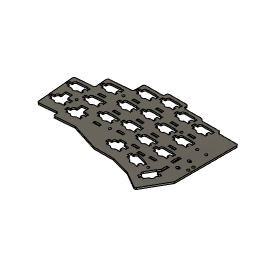
BottomCutout (Autodesk Fusion 360 design; units mm, degrees)
Autodesk Fusion 360 part; units mm, degrees
sketch "bottom-cutout-Edge_Cuts" plane through (0, 0, 0) normal (0, 0, 1) x (1, 0, 0)
  line L0 (132.25, -118) -> (132.25, -116)
  line L1 (110.25, -54.5) -> (110.25, -56.5)
  line L2 (121.75, -51.75) -> (124.5, -51.75)
  line L3 (121.75, -54.5) -> (121.75, -51.75)
  line L4 (130.75, -110.5) -> (130.75, -110)
  line L5 (140.75, -53.5) -> (140.75, -53)
  line L6 (126.75, -59) -> (129.25, -59)
  arc A0 (131.464, -53) -> (129.4503, -54.9213) centre (131.464, -55.016) ccw
  line L7 (121.75, -86.5) -> (112.464, -86.5)
  line L8 (123.25, -92.5) -> (121.75, -92.5)
  line L9 (129.45, -56) -> (129.45, -54.9321)
  line L10 (121.75, -92.5) -> (121.75, -89.75)
  line L11 (110.45, -89.5) -> (110.45, -88.4314)
  line L12 (129.25, -59) -> (129.25, -61)
  arc A1 (70.6704, -64.8002) -> (68.832, -66.8948) centre (70.8461, -66.8085) ccw
  line L13 (140.75, -53) -> (131.464, -53)
  arc A2 (73.5435, -72.8271) -> (77.7738, -72.457) centre (75.55, -71.4) ccw
  line L14 (66.2356, -68.1996) -> (66.4971, -71.1882)
  line L15 (142.25, -61) -> (142.25, -59)
  line L16 (124.5, -87) -> (121.75, -87)
  arc A3 (133.6268, -61.2468) -> (137.8732, -61.2468) centre (135.75, -60) ccw
  line L17 (123.25, -94.5) -> (123.25, -92.5)
  line L18 (140.75, -59) -> (140.75, -56.25)
  line L19 (143.5, -56.25) -> (143.5, -53.5)
  line L20 (138.3044, -61) -> (142.25, -61)
  line L21 (124.5, -89.75) -> (124.5, -87)
  line L22 (119.361, -94.5) -> (123.25, -94.5)
  line L23 (129.45, -56) -> (126.75, -56)
  line L24 (107.75, -92.5) -> (110.25, -92.5)
  line L25 (142.25, -59) -> (140.75, -59)
  line L26 (121.75, -89.75) -> (124.5, -89.75)
  line L27 (110.45, -89.5) -> (107.75, -89.5)
  line L28 (140.75, -56.25) -> (143.5, -56.25)
  line L29 (143.5, -53.5) -> (140.75, -53.5)
  line L30 (110.25, -94.5) -> (114.139, -94.5)
  line L31 (110.25, -56.5) -> (114.139, -56.5)
  arc A4 (114.6506, -94.7865) -> (118.8494, -94.7865) centre (116.75, -93.5) ccw
  line L32 (110.45, -51.5) -> (110.45, -50.4314)
  line L33 (124.5, -51.75) -> (124.5, -49)
  line L34 (119.45, -113) -> (116.75, -113)
  line L35 (116.75, -113) -> (116.75, -116)
  arc A5 (123.6268, -118.2468) -> (127.8732, -118.2468) centre (125.75, -117) ccw
  line L36 (133.5, -113.25) -> (133.5, -110.5)
  line L37 (121.75, -48.5) -> (112.464, -48.5)
  line L38 (128.3044, -118) -> (132.25, -118)
  line L39 (110.45, -51.5) -> (107.75, -51.5)
  line L40 (124.5, -49) -> (121.75, -49)
  line L41 (123.25, -56.5) -> (123.25, -54.5)
  line L42 (121.75, -87) -> (121.75, -86.5)
  line L43 (130.75, -116) -> (130.75, -113.25)
  line L44 (119.25, -118) -> (123.1956, -118)
  line L45 (119.25, -116) -> (119.25, -118)
  line L46 (133.5, -110.5) -> (130.75, -110.5)
  line L47 (132.25, -116) -> (130.75, -116)
  arc A6 (112.464, -86.5) -> (110.4502, -88.4221) centre (112.464, -88.516) ccw
  line L48 (107.75, -89.5) -> (107.75, -92.5)
  line L49 (130.75, -113.25) -> (133.5, -113.25)
  line L50 (119.45, -113) -> (119.45, -111.9321)
  arc A7 (121.464, -110) -> (119.4503, -111.9213) centre (121.464, -112.016) ccw
  line L51 (116.75, -116) -> (119.25, -116)
  line L52 (123.25, -54.5) -> (121.75, -54.5)
  line L53 (107.75, -51.5) -> (107.75, -54.5)
  arc A8 (112.464, -48.5) -> (110.4502, -50.4221) centre (112.464, -50.516) ccw
  line L54 (107.75, -54.5) -> (110.25, -54.5)
  line L55 (121.75, -49) -> (121.75, -48.5)
  arc A9 (114.6506, -56.7865) -> (118.8494, -56.7865) centre (116.75, -55.5) ccw
  line L56 (119.361, -56.5) -> (123.25, -56.5)
  line L57 (138.565, -116.455) -> (140.98, -117.102)
  line L58 (139.342, -113.557) -> (138.565, -116.455)
  line L59 (68.9253, -67.9643) -> (66.2356, -68.1996)
  line L60 (152.088, -120.078) -> (152.8, -117.422)
  line L61 (141.95, -114.256) -> (142.2254, -113.2276)
  line L62 (82.1124, -71.8297) -> (81.9381, -69.8373)
  line L63 (153.641, -114.283) -> (144.6718, -111.8797)
  line L64 (80.2041, -67.2285) -> (82.9437, -66.9888)
  line L65 (140.463, -119.034) -> (144.274, -120.0552)
  arc A10 (144.6265, -120.4051) -> (148.7284, -121.5036) centre (147, -119.75) ccw
  line L66 (78.1818, -72.1736) -> (82.1124, -71.8297)
  line L67 (152.8, -117.422) -> (155.456, -118.134)
  line L68 (79.9645, -64.489) -> (79.9209, -63.9909)
  line L69 (68.9253, -67.9643) -> (68.8326, -66.9036)
  line L70 (156.168, -115.477) -> (153.512, -114.766)
  arc A11 (75.1935, -91.7771) -> (79.4238, -91.407) centre (77.2, -90.35) ccw
  line L71 (141.95, -114.256) -> (139.342, -113.557)
  line L72 (140.98, -117.102) -> (140.463, -119.034)
  line L73 (81.9381, -69.8373) -> (80.4438, -69.968)
  line L74 (69.1619, -72.9627) -> (73.0925, -72.6188)
  line L75 (110.25, -92.5) -> (110.25, -94.5)
  line L76 (82.9437, -66.9888) -> (82.704, -64.2493)
  line L77 (153.537, -120.466) -> (152.088, -120.078)
  line L78 (129.25, -61) -> (133.1956, -61)
  line L79 (155.456, -118.134) -> (156.168, -115.477)
  arc A12 (144.6718, -111.8797) -> (142.2284, -113.2175) centre (144.15, -113.827) ccw
  line L80 (126.75, -56) -> (126.75, -59)
  line L81 (91.45, -74.5) -> (91.45, -73.4365)
  line L82 (104.25, -77.5) -> (102.75, -77.5)
  line L83 (102.75, -72) -> (102.75, -71.5)
  line L84 (88.75, -74.5) -> (88.75, -77.5)
  line L85 (100.3044, -79.5) -> (104.25, -79.5)
  line L86 (91.25, -77.5) -> (91.25, -79.5)
  arc A13 (93.4642, -71.5) -> (91.4502, -73.4263) centre (93.4642, -73.516) ccw
  line L87 (62.0819, -106.3735) -> (66.0124, -106.03)
  line L88 (50.1356, -102.4) -> (50.3971, -105.388)
  arc A14 (95.6268, -79.7468) -> (99.8732, -79.7468) centre (97.75, -78.5) ccw
  line L89 (63.8645, -98.689) -> (63.8209, -98.1909)
  line L90 (105.5, -74.75) -> (105.5, -72)
  line L91 (66.604, -98.4493) -> (63.8645, -98.689)
  line L92 (91.25, -79.5) -> (95.1956, -79.5)
  line L93 (51.1253, -83.1643) -> (48.4356, -83.3996)
  line L94 (104.25, -79.5) -> (104.25, -77.5)
  line L95 (102.75, -71.5) -> (93.4642, -71.5)
  arc A15 (54.5221, -99.0045) -> (52.7321, -101.0967) centre (54.7461, -101.008) ccw
  line L96 (66.8437, -101.189) -> (66.604, -98.4493)
  line L97 (88.75, -77.5) -> (91.25, -77.5)
  line L98 (66.0124, -106.03) -> (65.8381, -104.037)
  line L99 (52.8876, -105.17) -> (53.0619, -107.163)
  line L100 (64.3438, -104.168) -> (64.1041, -101.428)
  line L101 (102.75, -77.5) -> (102.75, -74.75)
  arc A16 (57.4434, -107.0269) -> (61.6738, -106.657) centre (59.45, -105.6) ccw
  line L102 (65.8381, -104.037) -> (64.3438, -104.168)
  line L103 (52.8254, -102.164) -> (52.7327, -101.1054)
  line L104 (50.3971, -105.388) -> (52.8876, -105.17)
  line L105 (91.45, -74.5) -> (88.75, -74.5)
  line L106 (48.4356, -83.3996) -> (48.6971, -86.3882)
  line L107 (60.4382, -87.3686) -> (64.3124, -87.0297)
  line L108 (62.6438, -85.168) -> (62.4041, -82.4285)
  line L109 (65.1437, -82.1888) -> (64.904, -79.4493)
  line L110 (105.5, -72) -> (102.75, -72)
  line L111 (102.75, -74.75) -> (105.5, -74.75)
  line L112 (70.6376, -89.9203) -> (70.8119, -91.9127)
  line L113 (68.1471, -90.1382) -> (70.6376, -89.9203)
  line L114 (81.5709, -82.9409) -> (72.3204, -83.7502)
  arc A17 (72.3204, -83.7502) -> (70.482, -85.8452) centre (72.4961, -85.7585) ccw
  line L115 (81.6145, -83.439) -> (81.5709, -82.9409)
  line L116 (67.8856, -87.1496) -> (68.1471, -90.1382)
  line L117 (83.5881, -88.7873) -> (82.0938, -88.918)
  line L118 (48.6971, -86.3882) -> (51.1876, -86.1703)
  line L119 (83.7624, -90.7797) -> (83.5881, -88.7873)
  line L120 (62.1209, -79.1909) -> (52.8704, -80.0002)
  arc A18 (52.8704, -80.0002) -> (51.0319, -82.094) centre (53.0461, -82.0085) ccw
  line L121 (64.1381, -85.0373) -> (62.6438, -85.168)
  line L122 (82.0938, -88.918) -> (81.8541, -86.1785)
  line L123 (64.904, -79.4493) -> (62.1645, -79.689)
  line L124 (70.5754, -86.9143) -> (67.8856, -87.1496)
  line L125 (70.5754, -86.9143) -> (70.4826, -85.8541)
  line L126 (81.8541, -86.1785) -> (84.5937, -85.9388)
  line L127 (62.4041, -82.4285) -> (65.1437, -82.1888)
  line L128 (51.1253, -83.1643) -> (51.0326, -82.1043)
  line L129 (79.8318, -91.1236) -> (83.7624, -90.7797)
  line L130 (62.1645, -79.689) -> (62.1209, -79.1909)
  line L131 (70.8119, -91.9127) -> (74.7425, -91.5688)
  arc A19 (55.7707, -88.0646) -> (59.9535, -87.6986) centre (57.75, -86.6) ccw
  line L132 (51.3619, -88.1627) -> (55.2361, -87.8238)
  line L133 (84.5937, -85.9388) -> (84.354, -83.1993)
  line L134 (64.3124, -87.0297) -> (64.1381, -85.0373)
  line L135 (84.354, -83.1993) -> (81.6145, -83.439)
  line L136 (66.4971, -71.1882) -> (68.9876, -70.9703)
  line L137 (80.4438, -69.968) -> (80.2041, -67.2285)
  line L138 (68.9876, -70.9703) -> (69.1619, -72.9627)
  line L139 (79.9209, -63.9909) -> (70.6704, -64.8002)
  line L140 (153.512, -114.766) -> (153.641, -114.283)
  line L141 (82.704, -64.2493) -> (79.9645, -64.489)
  line L142 (153.02, -122.398) -> (153.537, -120.466)
  line L143 (149.2088, -121.3767) -> (153.02, -122.398)
  line L144 (51.1876, -86.1703) -> (51.3619, -88.1627)
  line L145 (141.75, -110.5) -> (147.75, -110.5)
  line L146 (100.75, -66.5) -> (94.75, -66.5)
  line L147 (80.7046, -97.0396) -> (74.7275, -97.5625)
  line L148 (132.75, -69.0483) -> (138.75, -69.0483)
  line L149 (74.7275, -97.5625) -> (75.1678, -102.5953)
  line L150 (61.4514, -93.3423) -> (55.4743, -93.8653)
  line L151 (138.75, -105.048) -> (132.75, -105.048)
  line L152 (132.75, -67.0483) -> (132.75, -69.0483)
  line L153 (141.75, -108.5) -> (141.75, -110.5)
  line L154 (167.95, -107.3) -> (169.95, -107.3)
  line L155 (55.4743, -93.8653) -> (55.9132, -98.8827)
  line L156 (138.75, -67.0483) -> (132.75, -67.0483)
  line L157 (132.75, -88.0483) -> (138.75, -88.0483)
  line L158 (119.75, -62.5) -> (113.75, -62.5)
  line L159 (61.8903, -98.3598) -> (61.4514, -93.3423)
  line L160 (94.75, -87.5) -> (100.75, -87.5)
  arc A20 (175.35, -104.55) -> (175.35, -102.15) centre (175.35, -103.35) ccw
  line L161 (94.75, -104.5) -> (94.75, -106.5)
  line L162 (94.75, -68.5) -> (100.75, -68.5)
  line L163 (100.75, -106.5) -> (100.75, -104.5)
  line L164 (151.75, -109) -> (157.75, -109)
  line L165 (94.75, -106.5) -> (100.75, -106.5)
  line L166 (100.75, -87.5) -> (100.75, -85.5)
  circle A21 centre (181.75, -95.25) radius 1.25
  line L167 (100.75, -104.5) -> (94.75, -104.5)
  line L168 (151.75, -88) -> (151.75, -90)
  line L169 (138.75, -86.0483) -> (132.75, -86.0483)
  line L170 (132.75, -86.0483) -> (132.75, -88.0483)
  line L171 (151.75, -107) -> (151.75, -109)
  line L172 (94.75, -85.5) -> (94.75, -87.5)
  line L173 (128.75, -107.5) -> (122.75, -107.5)
  line L174 (173.366, -118.371) -> (171.634, -117.371)
  line L175 (163.884, -130.794) -> (165.134, -128.629)
  line L176 (138.75, -88.0483) -> (138.75, -86.0483)
  line L177 (128.75, -110) -> (128.75, -107.5)
  line L178 (157.75, -90) -> (157.75, -88)
  line L179 (151.75, -90) -> (157.75, -90)
  line L180 (122.75, -107.5) -> (122.75, -110)
  line L181 (119.75, -102.5) -> (119.75, -100.5)
  line L182 (113.75, -62.5) -> (113.75, -64.5)
  line L183 (151.75, -71) -> (157.75, -71)
  line L184 (157.75, -71) -> (157.75, -69)
  line L185 (157.75, -109) -> (157.75, -107)
  line L186 (119.75, -64.5) -> (119.75, -62.5)
  line L187 (157.75, -107) -> (151.75, -107)
  line L188 (113.75, -64.5) -> (119.75, -64.5)
  line L189 (157.75, -88) -> (151.75, -88)
  line L190 (157.75, -69) -> (151.75, -69)
  line L191 (151.75, -69) -> (151.75, -71)
  line L192 (170.884, -118.67) -> (168.502, -117.295)
  line L193 (168.502, -117.295) -> (169.95, -114.7865)
  line L194 (100.361, -60.5) -> (104.25, -60.5)
  line L195 (119.75, -100.5) -> (113.75, -100.5)
  line L196 (88.75, -58.5) -> (91.25, -58.5)
  line L197 (167.95, -112.7515) -> (166.121, -115.92)
  line L198 (79.223, -80.1043) -> (79.0487, -78.1119)
  line L199 (91.45, -93.5) -> (91.45, -92.4358)
  line L200 (104.25, -60.5) -> (104.25, -58.5)
  line L201 (102.75, -96.5) -> (102.75, -93.75)
  line L202 (91.45, -55.5) -> (91.45, -54.4358)
  line L203 (165.688, -115.67) -> (161.045, -123.712)
  line L204 (161.286, -129.294) -> (163.884, -130.794)
  line L205 (166.121, -115.92) -> (165.688, -115.67)
  arc A22 (95.6506, -60.7865) -> (99.8494, -60.7865) centre (97.75, -59.5) ccw
  line L206 (91.45, -93.5) -> (88.75, -93.5)
  line L207 (102.75, -53) -> (102.75, -52.5)
  line L208 (102.75, -55.75) -> (105.5, -55.75)
  line L209 (113.75, -100.5) -> (113.75, -102.5)
  line L210 (171.634, -117.371) -> (170.884, -118.67)
  line L211 (113.75, -83.5) -> (119.75, -83.5)
  line L212 (79.0487, -78.1119) -> (73.0715, -78.6348)
  line L213 (166.866, -129.629) -> (168.8391, -126.2121)
  line L214 (119.75, -83.5) -> (119.75, -81.5)
  line L215 (105.5, -93.75) -> (105.5, -91)
  line L216 (113.75, -81.5) -> (113.75, -83.5)
  line L217 (104.25, -98.5) -> (104.25, -96.5)
  line L218 (100.361, -98.5) -> (104.25, -98.5)
  line L219 (91.25, -98.5) -> (95.139, -98.5)
  line L220 (119.75, -81.5) -> (113.75, -81.5)
  line L221 (113.75, -102.5) -> (119.75, -102.5)
  line L222 (171.3931, -121.7876) -> (173.366, -118.371)
  line L223 (162.636, -126.956) -> (161.286, -129.294)
  line L224 (102.75, -58.5) -> (102.75, -55.75)
  line L225 (102.75, -52.5) -> (93.4642, -52.5)
  line L226 (88.75, -55.5) -> (88.75, -58.5)
  line L227 (104.25, -58.5) -> (102.75, -58.5)
  line L228 (73.0715, -78.6348) -> (73.2458, -80.6272)
  line L229 (73.2458, -80.6272) -> (79.223, -80.1043)
  line L230 (102.75, -90.5) -> (93.4642, -90.5)
  line L231 (91.45, -55.5) -> (88.75, -55.5)
  line L232 (91.25, -58.5) -> (91.25, -60.5)
  arc A23 (161.045, -123.712) -> (161.7079, -126.4203) centre (162.7911, -124.7199) ccw
  line L233 (105.5, -55.75) -> (105.5, -53)
  line L234 (105.5, -53) -> (102.75, -53)
  line L235 (102.75, -93.75) -> (105.5, -93.75)
  line L236 (91.25, -96.5) -> (91.25, -98.5)
  line L237 (165.134, -128.629) -> (166.866, -129.629)
  arc A24 (169.2683, -125.9621) -> (171.3913, -122.2845) centre (169.25, -123.5) ccw
  line L238 (104.25, -96.5) -> (102.75, -96.5)
  arc A25 (95.6506, -98.7865) -> (99.8494, -98.7865) centre (97.75, -97.5) ccw
  line L239 (105.5, -91) -> (102.75, -91)
  line L240 (162.636, -126.956) -> (161.7165, -126.4255)
  line L241 (91.25, -60.5) -> (95.139, -60.5)
  arc A26 (93.4642, -52.5) -> (91.4502, -54.427) centre (93.4642, -54.516) ccw
  line L242 (86.004, -102.149) -> (83.2645, -102.389)
  line L243 (159.75, -74) -> (150.464, -74)
  line L244 (88.75, -93.5) -> (88.75, -96.5)
  line L245 (148.25, -82) -> (152.139, -82)
  line L246 (143.5, -94.25) -> (143.5, -91.5)
  arc A27 (93.4642, -90.5) -> (91.4502, -92.427) centre (93.4642, -92.516) ccw
  line L247 (140.75, -91) -> (131.464, -91)
  arc A28 (133.6506, -99.2865) -> (137.8494, -99.2865) centre (135.75, -98) ccw
  arc A29 (152.6506, -82.2865) -> (156.8494, -82.2865) centre (154.75, -81) ccw
  line L248 (148.25, -80) -> (148.25, -82)
  line L249 (143.5, -91.5) -> (140.75, -91.5)
  line L250 (159.75, -61) -> (159.75, -58.25)
  line L251 (148.25, -63) -> (152.139, -63)
  arc A30 (76.8434, -110.7269) -> (81.0738, -110.357) centre (78.85, -109.3) ccw
  line L252 (72.4619, -110.863) -> (76.3923, -110.5186)
  line L253 (69.5356, -106.1) -> (69.7971, -109.088)
  arc A31 (73.9307, -102.7036) -> (72.132, -104.7955) centre (74.1461, -104.708) ccw
  line L254 (145.75, -80) -> (148.25, -80)
  line L255 (161.25, -80) -> (159.75, -80)
  arc A32 (131.464, -91) -> (129.4502, -92.9221) centre (131.464, -93.016) ccw
  line L256 (148.25, -61) -> (148.25, -63)
  line L257 (148.45, -77) -> (145.75, -77)
  line L258 (129.45, -94) -> (126.75, -94)
  line L259 (129.45, -94) -> (129.45, -92.9314)
  line L260 (159.75, -74.5) -> (159.75, -74)
  line L261 (140.75, -91.5) -> (140.75, -91)
  line L262 (159.75, -77.25) -> (162.5, -77.25)
  line L263 (69.7971, -109.088) -> (72.2876, -108.87)
  line L264 (86.2437, -104.889) -> (86.004, -102.149)
  line L265 (83.2645, -102.389) -> (83.2209, -101.891)
  line L266 (161.25, -82) -> (161.25, -80)
  line L267 (159.75, -58.25) -> (162.5, -58.25)
  line L268 (140.75, -78) -> (140.75, -75.25)
  line L269 (140.75, -97) -> (140.75, -94.25)
  line L270 (148.45, -58) -> (145.75, -58)
  line L271 (162.5, -74.5) -> (159.75, -74.5)
  line L272 (148.45, -58) -> (148.45, -56.9314)
  arc A33 (150.464, -74) -> (148.4502, -75.9221) centre (150.464, -76.016) ccw
  line L273 (72.2876, -108.87) -> (72.4619, -110.863)
  line L274 (157.361, -82) -> (161.25, -82)
  line L275 (129.25, -99) -> (133.139, -99)
  line L276 (159.75, -80) -> (159.75, -77.25)
  line L277 (126.75, -94) -> (126.75, -97)
  line L278 (142.25, -97) -> (140.75, -97)
  line L279 (88.75, -96.5) -> (91.25, -96.5)
  line L280 (83.5041, -105.128) -> (86.2437, -104.889)
  line L281 (145.75, -77) -> (145.75, -80)
  line L282 (83.7438, -107.868) -> (83.5041, -105.128)
  line L283 (85.2381, -107.737) -> (83.7438, -107.868)
  line L284 (138.361, -99) -> (142.25, -99)
  line L285 (162.5, -77.25) -> (162.5, -74.5)
  line L286 (129.25, -97) -> (129.25, -99)
  line L287 (142.25, -99) -> (142.25, -97)
  line L288 (126.75, -97) -> (129.25, -97)
  line L289 (140.75, -94.25) -> (143.5, -94.25)
  line L290 (72.2253, -105.864) -> (72.1327, -104.8056)
  line L291 (148.45, -77) -> (148.45, -75.9314)
  line L292 (159.75, -55) -> (150.464, -55)
  line L293 (85.4124, -109.73) -> (85.2381, -107.737)
  line L294 (81.4819, -110.0735) -> (85.4124, -109.73)
  line L295 (72.2253, -105.864) -> (69.5356, -106.1)
  line L296 (102.75, -91) -> (102.75, -90.5)
  line L297 (148.45, -96) -> (145.75, -96)
  line L298 (143.5, -72.5) -> (140.75, -72.5)
  line L299 (124.5, -68) -> (121.75, -68)
  line L300 (110.45, -70.5) -> (110.45, -69.4314)
  line L301 (145.75, -96) -> (145.75, -99)
  line L302 (121.75, -67.5) -> (112.464, -67.5)
  arc A34 (114.6506, -75.7865) -> (118.8494, -75.7865) centre (116.75, -74.5) ccw
  line L303 (140.75, -72.5) -> (140.75, -72)
  line L304 (140.75, -72) -> (131.464, -72)
  line L305 (148.45, -96) -> (148.45, -94.9314)
  line L306 (159.75, -99) -> (159.75, -96.25)
  arc A35 (112.464, -67.5) -> (110.4502, -69.4221) centre (112.464, -69.516) ccw
  arc A36 (150.464, -55) -> (148.4502, -56.9221) centre (150.464, -57.016) ccw
  line L307 (129.25, -78) -> (129.25, -80)
  line L308 (143.5, -75.25) -> (143.5, -72.5)
  line L309 (148.25, -101) -> (152.139, -101)
  line L310 (123.25, -73.5) -> (121.75, -73.5)
  line L311 (145.75, -99) -> (148.25, -99)
  arc A37 (152.6506, -63.2865) -> (156.8494, -63.2865) centre (154.75, -62) ccw
  line L312 (157.361, -101) -> (161.25, -101)
  line L313 (148.25, -99) -> (148.25, -101)
  line L314 (142.25, -80) -> (142.25, -78)
  line L315 (110.45, -70.5) -> (107.75, -70.5)
  line L316 (121.75, -70.75) -> (124.5, -70.75)
  line L317 (142.25, -78) -> (140.75, -78)
  line L318 (162.5, -58.25) -> (162.5, -55.5)
  line L319 (107.75, -73.5) -> (110.25, -73.5)
  line L320 (162.5, -96.25) -> (162.5, -93.5)
  line L321 (53.0619, -107.163) -> (56.9923, -106.8186)
  arc A38 (133.6506, -80.2865) -> (137.8494, -80.2865) centre (135.75, -79) ccw
  line L322 (119.361, -75.5) -> (123.25, -75.5)
  line L323 (129.25, -80) -> (133.139, -80)
  arc A39 (152.6506, -101.2865) -> (156.8494, -101.2865) centre (154.75, -100) ccw
  line L324 (145.75, -61) -> (148.25, -61)
  line L325 (138.361, -80) -> (142.25, -80)
  line L326 (129.45, -75) -> (129.45, -73.9314)
  line L327 (110.25, -73.5) -> (110.25, -75.5)
  line L328 (159.75, -55.5) -> (159.75, -55)
  line L329 (162.5, -55.5) -> (159.75, -55.5)
  line L330 (145.75, -58) -> (145.75, -61)
  line L331 (121.75, -73.5) -> (121.75, -70.75)
  line L332 (124.5, -70.75) -> (124.5, -68)
  line L333 (110.25, -75.5) -> (114.139, -75.5)
  line L334 (157.361, -63) -> (161.25, -63)
  line L335 (159.75, -93.5) -> (159.75, -93)
  line L336 (52.8254, -102.164) -> (50.1356, -102.4)
  line L337 (161.25, -101) -> (161.25, -99)
  line L338 (140.75, -75.25) -> (143.5, -75.25)
  line L339 (159.75, -93) -> (150.464, -93)
  line L340 (161.25, -99) -> (159.75, -99)
  line L341 (107.75, -70.5) -> (107.75, -73.5)
  line L342 (121.75, -68) -> (121.75, -67.5)
  line L343 (64.1041, -101.428) -> (66.8437, -101.189)
  line L344 (126.75, -75) -> (126.75, -78)
  line L345 (161.25, -63) -> (161.25, -61)
  arc A40 (150.464, -93) -> (148.4502, -94.9221) centre (150.464, -95.016) ccw
  line L346 (161.25, -61) -> (159.75, -61)
  line L347 (129.45, -75) -> (126.75, -75)
  line L348 (126.75, -78) -> (129.25, -78)
  line L349 (123.25, -75.5) -> (123.25, -73.5)
  line L350 (159.75, -96.25) -> (162.5, -96.25)
  line L351 (162.5, -93.5) -> (159.75, -93.5)
  arc A41 (131.464, -72) -> (129.4502, -73.9221) centre (131.464, -74.016) ccw
  line L352 (171.2979, -140.4529) -> (184.75, -117)
  line L353 (126.75, -48.5) -> (126.75, -47)
  arc A42 (69.3738, -116.3496) -> (67.7866, -114.9968) centre (67.8807, -116.494) ccw
  arc A43 (126.75, -47) -> (125.25, -45.5) centre (125.25, -47) ccw
  line L354 (89.25, -49.5) -> (105.25, -49.5)
  line L355 (86.288, -60.3907) -> (66.1036, -62.1006)
  line L356 (64.7491, -63.7144) -> (65.6216, -74.1884)
  line L357 (169.2522, -141.0013) -> (153.75, -132)
  circle A44 centre (181.75, -100.25) radius 1.25
  arc A45 (145.75, -51) -> (144.25, -50) centre (144.25, -51.625) ccw
  line L358 (174.15, -102.15) -> (175.35, -102.15)
  line L359 (125.25, -45.5) -> (108.25, -45.5)
  line L360 (174.15, -93.35) -> (175.35, -93.35)
  line L361 (128.25, -50) -> (144.25, -50)
  line L362 (168.5, -101.5) -> (166, -101.5)
  line L363 (135.3, -127) -> (116.25, -127)
  arc A46 (174.15, -102.15) -> (174.15, -104.55) centre (174.15, -103.35) ccw
  arc A47 (164.75, -53.25) -> (163.25, -52) centre (163.25, -53.525) ccw
  line L364 (64.2789, -75.7974) -> (48.2528, -77.2764)
  line L365 (168.5, -94) -> (168.5, -101.5)
  arc A48 (175.35, -93.35) -> (175.35, -90.95) centre (175.35, -92.15) ccw
  arc A49 (184.75, -56) -> (183.25, -54.5) centre (183.25, -56) ccw
  line L366 (166, -94) -> (168.5, -94)
  line L367 (183.25, -54.5) -> (166.25, -54.5)
  circle A50 centre (87.05, -69) radius 1.15
  line L368 (94.75, -66.5) -> (94.75, -68.5)
  line L369 (147.75, -108.5) -> (141.75, -108.5)
  line L370 (174.15, -104.55) -> (175.35, -104.55)
  arc A51 (69.5512, -118.8107) -> (70.9203, -120.0986) centre (70.9992, -118.643) ccw
  arc A52 (174.15, -90.95) -> (174.15, -93.35) centre (174.15, -92.15) ccw
  line L371 (174.15, -90.95) -> (175.35, -90.95)
  arc A53 (169.2541, -141.0024) -> (171.2967, -140.455) centre (170, -139.701) ccw
  line L372 (147.75, -110.5) -> (147.75, -108.5)
  line L373 (147.25, -52) -> (163.25, -52)
  circle A54 centre (108.25, -103.5) radius 1.15
  line L374 (46.9043, -78.8946) -> (50.125, -115.082)
  circle A55 centre (159.75, -117.5) radius 1.15
  line L375 (106.75, -47) -> (106.75, -48)
  line L376 (184.75, -87) -> (184.75, -117)
  line L377 (169.95, -107.3) -> (169.95, -114.7865)
  line L378 (167.95, -112.7515) -> (167.95, -107.3)
  line L379 (100.75, -85.5) -> (94.75, -85.5)
  circle A56 centre (67.5, -95.25) radius 1.15
  arc A57 (89.25, -49.5) -> (87.75, -51) centre (89.25, -51) ccw
  circle A58 centre (146.25, -71.5) radius 1.15
  line L380 (100.75, -68.5) -> (100.75, -66.5)
  arc A59 (145.75, -51) -> (147.25, -52) centre (147.25, -50.375) ccw
  line L381 (132.75, -105.048) -> (132.75, -107.048)
  line L382 (138.75, -107.048) -> (138.75, -105.048)
  line L383 (51.7337, -116.4465) -> (67.7757, -114.9977)
  circle A60 centre (168.75, -78.5) radius 1.15
  arc A61 (48.2497, -77.2767) -> (46.9041, -78.8919) centre (48.3991, -78.7693) ccw
  circle A62 centre (177.5, -78.5) radius 1.15
  line L384 (166, -101.5) -> (166, -94)
  line L385 (69.3747, -116.3594) -> (69.5495, -118.7934)
  line L386 (81.1449, -102.0726) -> (80.7046, -97.0396)
  line L387 (138.75, -69.0483) -> (138.75, -67.0483)
  line L388 (132.75, -107.048) -> (138.75, -107.048)
  arc A63 (126.75, -48.5) -> (128.25, -50) centre (128.25, -48.5) ccw
  arc A64 (64.2839, -75.7969) -> (65.6218, -74.1912) centre (64.126, -74.3051) ccw
  line L389 (184.75, -87) -> (184.75, -56)
  arc A65 (66.0984, -62.1011) -> (64.749, -63.7128) centre (66.2444, -63.5941) ccw
  arc A66 (86.31, -60.3883) -> (87.75, -58.75) centre (86.098, -58.75) ccw
  line L390 (135.3, -127) -> (153.75, -132)
  arc A67 (164.75, -53.25) -> (166.25, -54.5) centre (166.25, -52.975) ccw
  arc A68 (108.25, -45.5) -> (106.75, -47) centre (108.25, -47) ccw
  line L391 (89.25, -118.5) -> (116.25, -127)
  line L392 (87.75, -51) -> (87.75, -58.75)
  line L393 (70.9768, -120.0977) -> (89.25, -118.5)
  arc A69 (50.125, -115.082) -> (51.7263, -116.4471) centre (51.6192, -114.951) ccw
  arc A70 (105.25, -49.5) -> (106.75, -48) centre (105.25, -48) ccw
  line L394 (63.8209, -98.1909) -> (61.8903, -98.3598)
  line L395 (55.9132, -98.8827) -> (54.5293, -99.0038)
  arc A71 (57.4434, -107.0269) -> (56.9923, -106.8186) centre (57.0359, -107.3167) ccw
  arc A72 (62.0819, -106.3735) -> (61.6738, -106.657) centre (62.1254, -106.8716) ccw
  arc A73 (54.5293, -99.0038) -> (54.5221, -99.0045) centre (54.5554, -99.3027) ccw
  arc A74 (52.7321, -101.0967) -> (52.7327, -101.1054) centre (52.9319, -101.0879) ccw
  line L396 (83.2209, -101.891) -> (81.1449, -102.0726)
  line L397 (75.1678, -102.5953) -> (73.9406, -102.7026)
  arc A75 (76.8434, -110.7269) -> (76.3923, -110.5186) centre (76.4359, -111.0167) ccw
  arc A76 (81.4819, -110.0735) -> (81.0738, -110.357) centre (81.5254, -110.5716) ccw
  arc A77 (73.9406, -102.7026) -> (73.9307, -102.7036) centre (73.9841, -103.2007) ccw
  arc A78 (72.132, -104.7955) -> (72.1327, -104.8056) centre (72.3618, -104.7856) ccw
  arc A79 (51.0319, -82.094) -> (51.0326, -82.1043) centre (51.2617, -82.0843) ccw
  arc A80 (55.7707, -88.0646) -> (55.2361, -87.8238) centre (55.2884, -88.4215) ccw
  arc A81 (60.4382, -87.3686) -> (59.9535, -87.6986) centre (60.4905, -87.9664) ccw
  arc A82 (75.1935, -91.7771) -> (74.7425, -91.5688) centre (74.7861, -92.0669) ccw
  arc A83 (79.8318, -91.1236) -> (79.4238, -91.407) centre (79.8754, -91.6217) ccw
  arc A84 (70.482, -85.8452) -> (70.4826, -85.8541) centre (70.6818, -85.8366) ccw
  arc A85 (73.5435, -72.8271) -> (73.0925, -72.6188) centre (73.1361, -73.1169) ccw
  arc A86 (78.1818, -72.1736) -> (77.7738, -72.457) centre (78.2254, -72.6717) ccw
  arc A87 (68.832, -66.8948) -> (68.8326, -66.9036) centre (69.0318, -66.8862) ccw
  arc A88 (95.6268, -79.7468) -> (95.1956, -79.5) centre (95.1956, -80) ccw
  arc A89 (100.3044, -79.5) -> (99.8732, -79.7468) centre (100.3044, -80) ccw
  arc A90 (91.4502, -73.4263) -> (91.45, -73.4365) centre (91.68, -73.4365) ccw
  arc A91 (95.6506, -98.7865) -> (95.139, -98.5) centre (95.139, -99.1) ccw
  arc A92 (100.361, -98.5) -> (99.8494, -98.7865) centre (100.361, -99.1) ccw
  arc A93 (91.4502, -92.427) -> (91.45, -92.4358) centre (91.65, -92.4358) ccw
  arc A94 (123.6268, -118.2468) -> (123.1956, -118) centre (123.1956, -118.5) ccw
  arc A95 (128.3044, -118) -> (127.8732, -118.2468) centre (128.3044, -118.5) ccw
  arc A96 (119.4503, -111.9213) -> (119.45, -111.9321) centre (119.68, -111.9321) ccw
  line L398 (130.75, -110) -> (128.75, -110)
  line L399 (122.75, -110) -> (121.464, -110)
  arc A97 (144.6265, -120.4051) -> (144.274, -120.0552) centre (144.1446, -120.5382) ccw
  arc A98 (149.2088, -121.3767) -> (148.7284, -121.5036) centre (149.0794, -121.8597) ccw
  arc A99 (142.2284, -113.2175) -> (142.2254, -113.2276) centre (142.4476, -113.2871) ccw
  arc A100 (169.2683, -125.9621) -> (168.8391, -126.2121) centre (169.2721, -126.4621) ccw
  arc A101 (171.3931, -121.7876) -> (171.3913, -122.2845) centre (171.8261, -122.0376) ccw
  arc A102 (161.7079, -126.4203) -> (161.7165, -126.4255) centre (161.8315, -126.2263) ccw
  arc A103 (152.6506, -101.2865) -> (152.139, -101) centre (152.139, -101.6) ccw
  arc A104 (157.361, -101) -> (156.8494, -101.2865) centre (157.361, -101.6) ccw
  arc A105 (148.4502, -94.9221) -> (148.45, -94.9314) centre (148.65, -94.9314) ccw
  arc A106 (133.6506, -99.2865) -> (133.139, -99) centre (133.139, -99.6) ccw
  arc A107 (138.361, -99) -> (137.8494, -99.2865) centre (138.361, -99.6) ccw
  arc A108 (129.4502, -92.9221) -> (129.45, -92.9314) centre (129.65, -92.9314) ccw
  arc A109 (114.6506, -94.7865) -> (114.139, -94.5) centre (114.139, -95.1) ccw
  arc A110 (119.361, -94.5) -> (118.8494, -94.7865) centre (119.361, -95.1) ccw
  arc A111 (110.4502, -88.4221) -> (110.45, -88.4314) centre (110.65, -88.4314) ccw
  arc A112 (114.6506, -75.7865) -> (114.139, -75.5) centre (114.139, -76.1) ccw
  arc A113 (119.361, -75.5) -> (118.8494, -75.7865) centre (119.361, -76.1) ccw
  arc A114 (110.4502, -69.4221) -> (110.45, -69.4314) centre (110.65, -69.4314) ccw
  arc A115 (95.6506, -60.7865) -> (95.139, -60.5) centre (95.139, -61.1) ccw
  arc A116 (100.361, -60.5) -> (99.8494, -60.7865) centre (100.361, -61.1) ccw
  arc A117 (91.4502, -54.427) -> (91.45, -54.4358) centre (91.65, -54.4358) ccw
  arc A118 (114.6506, -56.7865) -> (114.139, -56.5) centre (114.139, -57.1) ccw
  arc A119 (119.361, -56.5) -> (118.8494, -56.7865) centre (119.361, -57.1) ccw
  arc A120 (110.4502, -50.4221) -> (110.45, -50.4314) centre (110.65, -50.4314) ccw
  arc A121 (133.6268, -61.2468) -> (133.1956, -61) centre (133.1956, -61.5) ccw
  arc A122 (138.3044, -61) -> (137.8732, -61.2468) centre (138.3044, -61.5) ccw
  arc A123 (129.4503, -54.9213) -> (129.45, -54.9321) centre (129.68, -54.9321) ccw
  arc A124 (152.6506, -63.2865) -> (152.139, -63) centre (152.139, -63.6) ccw
  arc A125 (157.361, -63) -> (156.8494, -63.2865) centre (157.361, -63.6) ccw
  arc A126 (148.4502, -56.9221) -> (148.45, -56.9314) centre (148.65, -56.9314) ccw
  arc A127 (133.6506, -80.2865) -> (133.139, -80) centre (133.139, -80.6) ccw
  arc A128 (138.361, -80) -> (137.8494, -80.2865) centre (138.361, -80.6) ccw
  arc A129 (129.4502, -73.9221) -> (129.45, -73.9314) centre (129.65, -73.9314) ccw
  arc A130 (152.6506, -82.2865) -> (152.139, -82) centre (152.139, -82.6) ccw
  arc A131 (157.361, -82) -> (156.8494, -82.2865) centre (157.361, -82.6) ccw
  arc A132 (148.4502, -75.9221) -> (148.45, -75.9314) centre (148.65, -75.9314) ccw
  arc A133 (70.9203, -120.0986) -> (70.9768, -120.0977) centre (70.9419, -119.6992) ccw
  arc A134 (69.5495, -118.7934) -> (69.5512, -118.8107) centre (69.9485, -118.7647) ccw
  arc A135 (69.3747, -116.3594) -> (69.3738, -116.3496) centre (68.9757, -116.3881) ccw
  arc A136 (67.7866, -114.9968) -> (67.7757, -114.9977) centre (67.8117, -115.3961) ccw
  arc A137 (51.7263, -116.4471) -> (51.7337, -116.4465) centre (51.6977, -116.0481) ccw
  arc A138 (46.9041, -78.8919) -> (46.9043, -78.8946) centre (47.3027, -78.8592) ccw
  arc A139 (48.2528, -77.2764) -> (48.2497, -77.2767) centre (48.2895, -77.6747) ccw
  arc A140 (65.6218, -74.1912) -> (65.6216, -74.1884) centre (65.2229, -74.2216) ccw
  arc A141 (64.749, -63.7128) -> (64.7491, -63.7144) centre (65.1478, -63.6812) ccw
  arc A142 (66.1036, -62.1006) -> (66.0984, -62.1011) centre (66.1374, -62.4992) ccw
  arc A143 (86.288, -60.3907) -> (86.31, -60.3883) centre (86.2458, -59.8925) ccw
  arc A144 (64.2789, -75.7974) -> (64.2839, -75.7969) centre (64.2445, -75.424) ccw
  arc A145 (169.2522, -141.0013) -> (169.2541, -141.0024) centre (169.453, -140.6554) ccw
  arc A146 (171.2967, -140.455) -> (171.2979, -140.4529) centre (170.9509, -140.2539) ccw
  dimension "d1" = 0.5
  dimension "d2" = 0.5
  dimension "d3" = 0.3
  dimension "d4" = 0.2
  dimension "d5" = 0.5
  dimension "d6" = 0.5
  dimension "d7" = 0.5
  dimension "d8" = 0.23
  dimension "d9" = 0.23
  dimension "d10" = 0.6
  dimension "d11" = 0.6
  dimension "d12" = 0.5
  dimension "d13" = 0.5
  dimension "d14" = 0.2
  dimension "d15" = 0.5
  dimension "d16" = 0.5
  dimension "d17" = 0.2
  dimension "d18" = 0.5
  dimension "d19" = 0.5
  dimension "d20" = 0.23
  dimension "d21" = 0.6
  dimension "d22" = 0.6
  dimension "d23" = 0.2
  dimension "d24" = 0.5
  dimension "d25" = 0.5
  dimension "d26" = 0.23
  dimension "d27" = 0.5
  dimension "d28" = 0.5
  dimension "d29" = 0.23
  dimension "d30" = 0.5
  dimension "d31" = 0.5
  dimension "d32" = 0.23
  dimension "d33" = 0.6
  dimension "d34" = 0.6
  dimension "d35" = 0.2
  dimension "d36" = 0.6
  dimension "d37" = 0.6
  dimension "d38" = 0.2
  dimension "d39" = 0.6
  dimension "d40" = 0.6
  dimension "d41" = 0.2
  dimension "d42" = 0.6
  dimension "d43" = 0.6
  dimension "d44" = 0.2
  dimension "d45" = 0.6
  dimension "d46" = 0.6
  dimension "d47" = 0.2
  dimension "d48" = 0.6
  dimension "d49" = 0.6
  dimension "d50" = 0.2
  dimension "d51" = 0.5
  dimension "d52" = 0.5
  dimension "d53" = 0.23
  dimension "d54" = 0.6
  dimension "d55" = 0.6
  dimension "d56" = 0.2
  dimension "d57" = 0.6
  dimension "d58" = 0.6
  dimension "d59" = 0.2
  dimension "d60" = 0.6
  dimension "d61" = 0.6
  dimension "d62" = 0.2
  dimension "d63" = 0.4
  dimension "d64" = 0.4
  dimension "d65" = 0.4
  dimension "d66" = 0.4
  dimension "d67" = 0.4
  dimension "d68" = 0.4
  dimension "d69" = 0.4
  dimension "d70" = 0.4
  dimension "d71" = 0.4
  dimension "d72" = 0.4
  dimension "d73" = 0.5
  dimension "d74" = 0.375
  dimension "d75" = 0.4
  dimension "d76" = 0.4
  constraint coincident L155.end L394
  constraint collinear L394 L395
  constraint tangent L321 A71
  constraint tangent A16 A71
  constraint tangent L87 A72
  constraint tangent A16 A72
  constraint tangent L395 A73
  constraint tangent A15 A73
  constraint tangent L103 A74
  constraint tangent A15 A74
  constraint coincident L149.end L396
  constraint collinear L396 L397
  constraint tangent L252 A75
  constraint tangent A30 A75
  constraint tangent L294 A76
  constraint tangent A30 A76
  constraint tangent L397 A77
  constraint tangent A31 A77
  constraint tangent L290 A78
  constraint tangent A31 A78
  constraint tangent L128 A79
  constraint tangent A18 A79
  constraint tangent L132 A80
  constraint tangent A19 A80
  constraint tangent A19 A81
  constraint tangent L107 A81
  constraint tangent L131 A82
  constraint tangent A11 A82
  constraint tangent L129 A83
  constraint tangent A11 A83
  constraint tangent L125 A84
  constraint tangent A17 A84
  constraint tangent L74 A85
  constraint tangent A2 A85
  constraint tangent L66 A86
  constraint tangent A2 A86
  constraint tangent L69 A87
  constraint tangent A1 A87
  constraint tangent L92 A88
  constraint tangent A14 A88
  constraint tangent A14 A89
  constraint tangent L85 A89
  constraint tangent L81 A90
  constraint tangent A13 A90
  constraint tangent L219 A91
  constraint tangent A25 A91
  constraint tangent L218 A92
  constraint tangent A25 A92
  constraint tangent L199 A93
  constraint tangent A27 A93
  constraint tangent L44 A94
  constraint tangent A5 A94
  constraint tangent L38 A95
  constraint tangent A5 A95
  constraint tangent L50 A96
  constraint tangent A7 A96
  constraint coincident L180.end L398
  constraint collinear L398 L399
  constraint tangent L65 A97
  constraint tangent A10 A97
  constraint tangent L143 A98
  constraint tangent A10 A98
  constraint tangent L61 A99
  constraint tangent A12 A99
  constraint tangent L213 A100
  constraint tangent A24 A100
  constraint tangent L222 A101
  constraint tangent A24 A101
  constraint tangent L240 A102
  constraint tangent A23 A102
  constraint tangent L309 A103
  constraint tangent A39 A103
  constraint tangent L312 A104
  constraint tangent A39 A104
  constraint tangent L305 A105
  constraint tangent A40 A105
  constraint tangent L275 A106
  constraint tangent A28 A106
  constraint tangent L284 A107
  constraint tangent A28 A107
  constraint tangent L259 A108
  constraint tangent A32 A108
  constraint tangent L30 A109
  constraint tangent A4 A109
  constraint tangent L22 A110
  constraint tangent A4 A110
  constraint tangent L11 A111
  constraint tangent A6 A111
  constraint tangent L333 A112
  constraint tangent A34 A112
  constraint tangent L322 A113
  constraint tangent A34 A113
  constraint tangent L300 A114
  constraint tangent A35 A114
  constraint tangent L241 A115
  constraint tangent A22 A115
  constraint tangent L194 A116
  constraint tangent A22 A116
  constraint tangent L202 A117
  constraint tangent A26 A117
  constraint tangent L31 A118
  constraint tangent A9 A118
  constraint tangent L56 A119
  constraint tangent A9 A119
  constraint tangent L32 A120
  constraint tangent A8 A120
  constraint tangent L78 A121
  constraint tangent A3 A121
  constraint tangent L20 A122
  constraint tangent A3 A122
  constraint tangent L9 A123
  constraint tangent A0 A123
  constraint tangent L251 A124
  constraint tangent A37 A124
  constraint tangent L334 A125
  constraint tangent A37 A125
  constraint tangent L272 A126
  constraint tangent A36 A126
  constraint tangent L323 A127
  constraint tangent A38 A127
  constraint tangent L325 A128
  constraint tangent A38 A128
  constraint tangent L326 A129
  constraint tangent A41 A129
  constraint tangent L245 A130
  constraint tangent A29 A130
  constraint tangent L274 A131
  constraint tangent A29 A131
  constraint tangent L291 A132
  constraint tangent A33 A132
  constraint tangent L393 A133
  constraint tangent A51 A133
  constraint tangent L385 A134
  constraint tangent A51 A134
  constraint tangent L385 A135
  constraint tangent A42 A135
  constraint tangent L383 A136
  constraint tangent A42 A136
  constraint tangent L383 A137
  constraint tangent A69 A137
  constraint tangent L374 A138
  constraint tangent A61 A138
  constraint tangent L364 A139
  constraint tangent A61 A139
  constraint tangent L356 A140
  constraint tangent A64 A140
  constraint tangent L356 A141
  constraint tangent A65 A141
  constraint tangent L355 A142
  constraint tangent A65 A142
  constraint tangent L355 A143
  constraint tangent A66 A143
  constraint tangent L364 A144
  constraint tangent A64 A144
  constraint tangent L357 A145
  constraint tangent A53 A145
  constraint tangent L352 A146
  constraint tangent A53 A146
  measures "d1" radius of A71
  measures "d2" radius of A72
  measures "d3" radius of A73
  measures "d4" radius of A74
  measures "d5" radius of A75
  measures "d6" radius of A76
  measures "d7" radius of A77
  measures "d8" radius of A78
  measures "d9" radius of A79
  measures "d10" radius of A80
  measures "d11" radius of A81
  measures "d12" radius of A82
  measures "d13" radius of A83
  measures "d14" radius of A84
  measures "d15" radius of A85
  measures "d16" radius of A86
  measures "d17" radius of A87
  measures "d18" radius of A88
  measures "d19" radius of A89
  measures "d20" radius of A90
  measures "d21" radius of A91
  measures "d22" radius of A92
  measures "d23" radius of A93
  measures "d24" radius of A94
  measures "d25" radius of A95
  measures "d26" radius of A96
  measures "d27" radius of A97
  measures "d28" radius of A98
  measures "d29" radius of A99
  measures "d30" radius of A100
  measures "d31" radius of A101
  measures "d32" radius of A102
  measures "d33" radius of A103
  measures "d34" radius of A104
  measures "d35" radius of A105
  measures "d36" radius of A106
  measures "d37" radius of A107
  measures "d38" radius of A108
  measures "d39" radius of A109
  measures "d40" radius of A110
  measures "d41" radius of A111
  measures "d42" radius of A112
  measures "d43" radius of A113
  measures "d44" radius of A114
  measures "d45" radius of A115
  measures "d46" radius of A116
  measures "d47" radius of A117
  measures "d48" radius of A118
  measures "d49" radius of A119
  measures "d50" radius of A120
  measures "d51" radius of A121
  measures "d52" radius of A122
  measures "d53" radius of A123
  measures "d54" radius of A124
  measures "d55" radius of A125
  measures "d56" radius of A126
  measures "d57" radius of A127
  measures "d58" radius of A128
  measures "d59" radius of A129
  measures "d60" radius of A130
  measures "d61" radius of A131
  measures "d62" radius of A132
  measures "d63" radius of A133
  measures "d64" radius of A134
  measures "d65" radius of A135
  measures "d66" radius of A136
  measures "d67" radius of A137
  measures "d68" radius of A138
  measures "d69" radius of A139
  measures "d70" radius of A140
  measures "d71" radius of A141
  measures "d72" radius of A142
  measures "d73" radius of A143
  measures "d74" radius of A144
  measures "d75" radius of A145
  measures "d76" radius of A146
extrude "Extrude1" add sketch "bottom-cutout-Edge_Cuts" along normal blind 1.5 contours A141 | L352 L353 A42 A43 L354 L355 L356 L357 A45 L359 L361 L363 A47 L364 A49 L367 A51 A53 L373 L374 L375 L376 A57 A59 L383 A61 L385 A63 A64 L389 A65 A66 L390 A67 A68 L391 L392 L393 A69 A70 A133 A134 A135 A136 A137 A138 A139 A140 A142 A143 A144 A146 | A145
